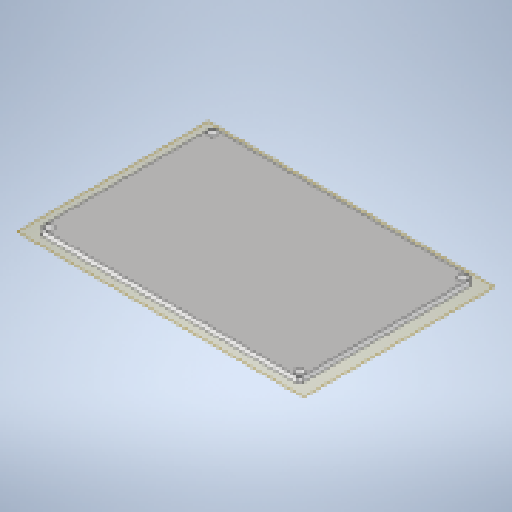
# Autodesk Inventor part: OCTOPUS_BOX_LID
Saved by Autodesk Inventor 2025.2 (Build 292293000, 293)
## iProperties
Created: 2026-03-26
Part Number: OCTOPUS_BOX_LID
Material: Generic
Document SubType Name: Modeling
Designer: composite
Density: 1 g/cm^3
Appearance: Default
Author: composite
Autodesk Inventor part; units mm, degrees
ref_plane "YZ Plane" through (0, 0, 0) normal (1, 0, 0) x (0, 1, 0)
ref_plane "XZ Plane" through (0, 0, 0) normal (0, 1, 0) x (-1, 0, 0)
ref_plane "XY Plane" through (0, 0, 0) normal (0, 0, 1) x (1, 0, 0)
ref_plane "Work Plane1" through (224.0032, 379.4573, 423.8682) normal (0, 1, 0) x (0, 0, 1)
sketch "Sketch1" plane through (224.0032, 379.4573, 423.8682) normal (0, 1, 0) x (0, 0, 1)
  circle A0 centre (56.5, 86.5) radius 3 projected
  circle A1 centre (-56.5, -86.5) radius 3 projected
  arc A2 (-60, -88) -> (-58, -90) centre (-58, -88) ccw projected
  line L0 (-58, -90) -> (58, -90) projected
  arc A3 (58, -90) -> (60, -88) centre (58, -88) ccw projected
  line L1 (60, -88) -> (60, 88) projected
  arc A4 (60, 88) -> (58, 90) centre (58, 88) ccw projected
  line L2 (58, 90) -> (-58, 90) projected
  arc A5 (-58, 90) -> (-60, 88) centre (-58, 88) ccw projected
  line L3 (-60, 88) -> (-60, -88) projected
  line L4 (54, 82) -> (54, -82) projected
  arc A6 (52, -84) -> (54, -82) centre (52, -82) ccw projected
  line L5 (52, -84) -> (-52, -84) projected
  arc A7 (-54, -82) -> (-52, -84) centre (-52, -82) ccw projected
  line L6 (-54, -82) -> (-54, 82) projected
  arc A8 (-52, 84) -> (-54, 82) centre (-52, 82) ccw projected
  line L7 (-52, 84) -> (52, 84) projected
  arc A9 (54, 82) -> (52, 84) centre (52, 82) ccw projected
  circle A10 centre (-56.5, 86.5) radius 3 projected
  circle A11 centre (56.5, -86.5) radius 3 projected
  point P0 (-423.8682, -224.0032)
extrude "Extrusion1" add sketch "Sketch1" along normal blind 4 contours L3 A5 L2 A4 L1 A3 L0 A2 | L4 A6 L5 A7 L6 A8 L7 A9
body "Solid1"
